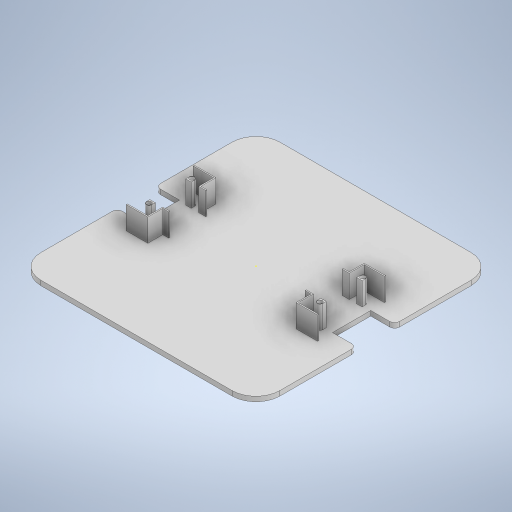
# Autodesk Inventor part: heheheha
Saved by Autodesk Inventor 2023 (Build 270158000, 158)
## iProperties
Created: 2022-12-15
Part Number: heheheha
Material: Ogólny
Document SubType Name: Modeling
Designer: User
Density: 1 g/cm^3
Appearance: Domyślna
Author: User
Autodesk Inventor part; units mm, degrees
ref_plane "YZ Plane" through (0, 0, 0) normal (1, 0, 0) x (0, 1, 0)
ref_plane "XZ Plane" through (0, 0, 0) normal (0, 1, 0) x (-1, 0, 0)
ref_plane "XY Plane" through (0, 0, 0) normal (0, 0, 1) x (1, 0, 0)
sketch "Szkic2" plane through (0, 0, 0) normal (0, 1, 0) x (-1, 0, 0)
  line L0 (50, -50) -> (-50, -50)
  line L1 (50, -50) -> (50, 50)
  line L2 (0, -53.6442) -> (0, 78.3558)
  line L3 (50, 50) -> (-50, 50)
  line L4 (-50, -50) -> (-50, 50)
  line L5 (67.5466, 0) -> (-74.1589, 0)
  line L6 (50, -8) -> (40, -8)
  line L7 (40, -8) -> (40, 8)
  line L8 (40, 8) -> (50, 8)
  line L9 (50, 8) -> (50, -8)
  line L10 (-50, -8) -> (-40, -8)
  line L11 (-40, -8) -> (-40, 8)
  line L12 (-40, 8) -> (-50, 8)
  line L13 (-50, 8) -> (-50, -8)
  line L14 (40, -7.5) -> (28.5, -7.5)
  line L15 (28.5, -7.5) -> (28.5, 7.5)
  line L16 (28.5, 7.5) -> (40, 7.5)
  line L17 (40, 7.5) -> (40, -7.5)
  line L18 (-40, -7.5) -> (-28.5, -7.5)
  line L19 (-28.5, -7.5) -> (-28.5, 7.5)
  line L20 (-28.5, 7.5) -> (-40, 7.5)
  line L21 (-40, 7.5) -> (-40, -7.5)
  line L22 (31.5, 8) -> (-31.5, 8)
  line L23 (28.5, 7.5) -> (28.5, 8)
  line L24 (-28.5, 7.5) -> (-28.5, 8)
  line L25 (31.5, -8) -> (-31.5, -8)
  line L26 (-28.5, -7.5) -> (-28.5, -8)
  line L27 (28.5, -7.5) -> (28.5, -8)
  line L28 (31.5, -8) -> (31.5, -13.75)
  line L29 (31.5, -13.75) -> (40, -13.75)
  line L30 (40, -13.75) -> (40, -8)
  line L31 (31.5, 8) -> (31.5, 13.75)
  line L32 (31.5, 13.75) -> (40, 13.75)
  line L33 (40, 13.75) -> (40, 8)
  line L34 (-31.5, -13.75) -> (-40, -13.75)
  line L35 (-40, -13.75) -> (-40, -8)
  line L36 (-31.5, -8) -> (-31.5, -13.75)
  line L37 (-31.5, 8) -> (-31.5, 13.75)
  line L38 (-31.5, 13.75) -> (-40, 13.75)
  line L39 (-40, 13.75) -> (-40, 8)
  circle A0 centre (35.75, -9) radius 1.15
  line L40 (40, -8) -> (40, -7.5)
  line L41 (31.5, -8) -> (31.5, -7.5)
  line L42 (-31.5, -8) -> (-31.5, -7.5)
  line L43 (-40, -8) -> (-40, -7.5)
  line L44 (40, 8) -> (40, 7.5)
  line L45 (31.5, 8) -> (31.5, 7.5)
  line L46 (-31.5, 8) -> (-31.5, 7.5)
  line L47 (-40, 8) -> (-40, 7.5)
  line L48 (40, -8) -> (40, -8)
  line L49 (40, 8) -> (40, 8)
  line L50 (-40, -8) -> (-40, -8)
  line L51 (-40, 8) -> (-40, 8)
  circle A1 centre (35.75, 9) radius 1.15
  circle A2 centre (-35.75, -9) radius 1.15
  circle A3 centre (-35.75, 9) radius 1.15
  circle A4 centre (35.75, -9) radius 1
  line L52 (36.9, -9) -> (36.9, -7.5)
  line L53 (34.6, -9) -> (34.6, -7.5)
  line L54 (31, -8) -> (31, -14.25)
  line L55 (31, -14.25) -> (40.0775, -14.25)
  line L56 (40, -14.25) -> (40, -13.75)
  circle A5 centre (35.75, 9) radius 1
  line L57 (36.9, 9) -> (36.9, 7.5)
  line L58 (34.6, 9) -> (34.6, 7.5)
  line L59 (31, 8) -> (31, 14.25)
  line L60 (31, 14.25) -> (40.0775, 14.25)
  line L61 (40, 14.25) -> (40, 13.75)
  circle A6 centre (-35.75, -9) radius 1.15
  circle A7 centre (-35.75, -9) radius 1
  line L62 (-36.9, -9) -> (-36.9, -7.5)
  line L63 (-34.6, -9) -> (-34.6, -7.5)
  circle A8 centre (-35.75, 9) radius 1.15
  circle A9 centre (-35.75, 9) radius 1
  line L64 (-36.9, 9) -> (-36.9, 7.5)
  line L65 (-34.6, 9) -> (-34.6, 7.5)
  line L66 (-31, -8) -> (-31, -14.9986)
  line L67 (-31, -14.25) -> (-40, -14.25)
  line L68 (-40, -14.25) -> (-40, -13.75)
  line L69 (-31, 8) -> (-31, 14.9986)
  line L70 (-31, 14.25) -> (-40, 14.25)
  line L71 (-40, 14.25) -> (-40, 13.75)
  line L72 (50, -50) -> (50, 50)
  line L73 (50, -50) -> (-50, -50)
  line L74 (50, -8) -> (40, -8)
  line L75 (40, 8) -> (50, 8)
  line L76 (40, 7.5) -> (40, -7.5)
  line L77 (50, -50) -> (-50, -50)
  line L78 (-40, 0) -> (-9.8, 0)
  line L79 (-9.7869, 8) -> (-9.7869, -8)
  line L80 (9.7869, 8) -> (9.7869, -8)
  point P0 (0, 0)
  point P1 (50, 8)
  point P2 (-50, 8)
  point P3 (-34.25, -7.5)
  point P4 (27.1, -10.7133)
  point P5 (21.7, -10.7133)
  point P6 (31.5, 8)
  point P7 (27.1, 10.7133)
  point P8 (40, 7.5)
  point P9 (-36.9, 9)
  point P10 (-36.9, 7.5)
  point P11 (-34.6, 7.5)
  point P12 (-31.5, 7.5)
  point P13 (-31, 8)
  point P14 (-36.9, -9)
  point P15 (-34.6, -7.5)
  point P16 (-36.9, -7.5)
  point P17 (-31.5, -7.5)
  point P18 (36.9, 9)
  point P19 (34.6, 7.5)
  point P20 (36.9, 7.5)
  point P21 (31, 8)
  point P22 (31.5, 7.5)
  point P23 (-50, 0)
  dimension "d30" = 100
  dimension "d31" = 132
  dimension "d32" = 16
  dimension "d33" = 10
  dimension "d38" = 11.5
  dimension "d39" = 15
  dimension "d40" = 15
  dimension "d41" = 11.5
  dimension "d42" = 10
  dimension "d44" = 15
  dimension "d47" = 0
  dimension "d48" = 3
  dimension "d49" = 5.75
  dimension "d50" = 2.3
  dimension "d56" = 2
  dimension "d59" = 3.1
  dimension "d60" = 0.5
  dimension "d61" = 0.5
  dimension "d62" = 0.5
  dimension "d63" = 0.5
  dimension "d68" = 100
  dimension "d69" = 50
  dimension "d70" = 30.2
  constraints: 158 end point, 40 symmetric about line, 20 point on line, 17 vertical, 15 horizontal, 13 parallel, 11 perpendicular, 10 centre point, 7 midpoint, 4 point on circle, 2 coincident, 2 tangent, 1 collinear, 72 other
  measures "d30" distance of L0.start L0.end
  measures "d31" distance of L2.start L2.end
  measures "d32" distance of L6.end L7.end
  measures "d33" distance of L6.start L6.end
  measures "d38" distance of L14.start L14.end
  measures "d39" distance of L14.end L15.end
  measures "d40" distance of L20.end L18.start
  measures "d41" distance of L18.start L18.end
  measures "d42" distance of L10.start L10.end
  measures "d44" distance from line of L20 point (-34.25, -7.5)
  measures "d47" distance of L6.end L40.start
  measures "d48" distance of L27.end L41.start
  measures "d49" distance of L41.start L28.end
  measures "d50" diameter of A0
  measures "d56" diameter of A4
  measures "d59" distance of L14.start L52.end
  measures "d60" distance between parallel lines of L54 L28
  measures "d61" distance between parallel lines of L29 L55
  measures "d62" distance of L34.end L67.end
  measures "d63" distance between parallel lines of L36 L66
  measures "d68" distance of L0.end L3.end
  measures "d69" distance of point (-50, 0) L3.end
  measures "d70" distance of L78.start L78.end
extrude "Wyciągnięcie proste3" add sketch "Szkic2" along normal blind 11.5 contours L56 L55 L54 L25 L28 L29 | L27 L14 L41 L25 | L25 L42 L18 L26 | L52 A0 L53 L14 | L34 L36 L25 L66 L67 L68 | L32 L31 L22 L59 L60 L61 | L23 L22 L45 L16 | L16 L58 A1 L57 | A0 | L18 L63 A2 L62 | L24 L20 L46 L22 | A1 | L71 L70 L69 L22 L37 L38 | L64 A3 L65 L20 | A2 | A3
extrude "Wyciągnięcie proste4" add sketch "Szkic2" along normal blind 2 separate body contours L0 L2 L25 L54 L55 L56 L30 L6 L1 | L0 L4 L10 L35 L68 L67 L66 L25 L2 | L25 L79 L5 L2 | L2 L5 L80 L25 | L30 L29 L28 L41 L14 L53 A0 L52 L7 | L5 L79 L22 L2 | L2 L22 L80 L5 | L80 L5 L15 L27 L25 | L25 L26 L19 L5 L79 | L8 L33 L61 L60 L59 L22 L2 L3 L1 | L7 L14 L15 L5 | L5 L15 L16 L7 | L11 L18 L62 A2 L63 L42 L36 L34 L35 | L22 L69 L70 L71 L39 L12 L4 L3 L2 | L80 L22 L23 L15 L5 | L5 L19 L24 L22 L79 | L7 L16 L57 A1 L58 L45 L31 L32 L33 | L11 L20 L19 L5 | L5 L19 L18 L11 | L39 L38 L37 L46 L20 L65 A3 L64 L11 | A4 | A5 | A7 | A9
fillet "Zaokrąglenie4" radius 10 4 edges at (-50, 1, -50) (-50, 1, 50) (50, 1, 50) (50, 1, -50)
fillet "Zaokrąglenie5" radius 2 4 edges at (50, 1, 8) (50, 1, -8) (-50, 1, 8) (-50, 1, -8)
sketch "Szkic3" plane through (0, 2, 0) normal (0, 1, 0) x (1, 0, 0)
  point P0 (0, 0)
